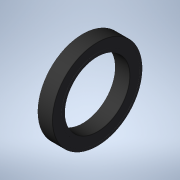
# Autodesk Inventor part: C-E6806ZZ
Saved by Autodesk Inventor 2021 (Build 250183000, 183)
## iProperties
Created: 2025-11-23
Part Number: C-E6806ZZ
Material: Generic
Catalog Web Link: www.3dfindit.com
Description: C-E6___ZZ-Economy Deep Groove Ball Bearing - Double Shielded, Single Row
Vendor: MISUMI
Document SubType Name: Modeling
Designer: psAdmin
Manufacturer: MISUMI
Mass: 4.68791 g
Surface Area: 29.1901 cm^2
Volume: 4.68791 cm^3
Density: 1 g/cm^3
Appearance: PSOLRGB-176-176-176
Category: PARTsolutions
Company: MISUMI
Title: C-E6806ZZ
Author: Cadenas PARTsolutions
Comments: Economy Deep Groove Ball Bearing - Double Shielded, Single Row
PSOL_IDENT_0: {$CADENAS_DATA/23d-libs/misumi/metric/12_bearing_holders/c_e6700zz.prj},162 {VTYP=3D},{NB=C-E6806ZZ}
PSOL_IDENT_1: ,{LINA=C-E6806ZZ},{NN=C-E6___ZZ},{DATE=29.05.2023 02:13:12},{GEOMDATE=25.05.2021 01:16:58},{VERSION=
PSOL_IDENT_2: },{LINEID=250},{WBVAR=},{WBNUMERIC=}  {NB=C-E6806ZZ},{LINA=C-E6806ZZ},{KT=DUMMY},{PN=C-E6806ZZ},{TS=
PSOL_IDENT_3: C-E6806ZZ},{DD=30},{D=42},{B=7},{RR=0.3},{AA=6.8390},{BB=1.3900},{CC=1.7000}
NB: C-E6806ZZ
NN: C-E6___ZZ
NT: Economy Deep Groove Ball Bearing - Double Shielded, Single Row
NBSYN: $PN.
LINA: C-E6806ZZ
CATALOG: Misumi
PN: C-E6806ZZ
TS: C-E6806ZZ
DD: 30
D: 42
B: 7
RR: 0.3
SUPPLIER: MISUMI
ARTICLENO: C-E6806ZZ
BOMINFO: C-E6806ZZ
CREATOR: CADENAS GmbH
Autodesk Inventor part; units mm, degrees
sketch "Sketch_1" plane through (0, 0, 0) normal (0, 0, 1) x (1, 0, 0)
  line L0 (7, 0) -> (0, 0)
  arc A0 (0, 15.3) -> (0.3, 15) centre (0.3, 15.3) ccw
  line L1 (0.3, 15) -> (6.7, 15)
  arc A1 (6.7, 15) -> (7, 15.3) centre (6.7, 15.3) ccw
  line L2 (7, 15.3) -> (7, 16.7)
  line L3 (7, 16.7) -> (6.9195, 16.7)
  line L4 (6.9195, 16.7) -> (6.9195, 19.61)
  line L5 (6.9195, 19.61) -> (7, 19.61)
  line L6 (7, 19.61) -> (7, 20.7)
  arc A2 (7, 20.7) -> (6.7, 21) centre (6.7, 20.7) ccw
  line L7 (6.7, 21) -> (0.3, 21)
  arc A3 (0.3, 21) -> (0, 20.7) centre (0.3, 20.7) ccw
  line L8 (0, 20.7) -> (0, 19.61)
  line L9 (0, 19.61) -> (0.0805, 19.61)
  line L10 (0.0805, 19.61) -> (0.0805, 16.7)
  line L11 (0.0805, 16.7) -> (0, 16.7)
  line L12 (0, 16.7) -> (0, 15.3)
  constraints: 26 end point, 8 point on circle, 4 centre point
revolve "Revolution1" add sketch "Sketch_1" angle 360 about axis through (7, 0, 0) along (1, 0, 0)
ref_plane "center_point_XY" through (3.5, 0, 0) normal (1, 0, 0) x (0, 0, -1)
ref_plane "center_point_YZ" through (3.5, 0, 0) normal (0, 0, -1) x (0, 1, 0)
ref_plane "center_point_ZX" through (3.5, 0, 0) normal (0, 1, 0) x (1, 0, 0)
ref_plane "to_housing_XY" through (0, 0, 0) normal (1, 0, 0) x (0, 0, -1)
ref_plane "to_housing_YZ" through (0, 0, 0) normal (0, 0, -1) x (0, 1, 0)
ref_plane "to_housing_ZX" through (0, 0, 0) normal (0, 1, 0) x (1, 0, 0)
ref_plane "to_ring_XY" through (6.839, 0, 0) normal (1, 0, 0) x (0, 0, -1)
ref_plane "to_ring_YZ" through (6.839, 0, 0) normal (0, 0, -1) x (0, 1, 0)
ref_plane "to_ring_ZX" through (6.839, 0, 0) normal (0, 1, 0) x (1, 0, 0)
body "Solid1"
